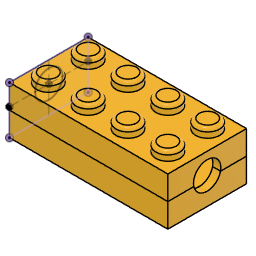
2x4 lego brick 3001 v6 v3 (Autodesk Fusion 360 design; units mm, degrees)
Autodesk Fusion 360 part; units mm, degrees
box "BoxPrimitive1" add length 15.8 width 31.8 height 9.6 placed x (0, 0, -1) y (-1, 0, 0) z (0, 1, 0) at (31.8, 0, 0) makes body 1
box "BoxPrimitive2" add length 13.4 width 29.4 height 8.6 placed x (0, 0, 1) y (1, 0, 0) z (0, 1, 0) at (0, 0, 0) separate body makes body 2
move_body "Move2" bodies 2 to x (1, 0, 0) y (0, 1, 0) z (0, 0, 1) at (1.2, 0, 0)
move_body "Move3" bodies 2 to x (1, 0, 0) y (0, 1, 0) z (0, 0, 1) at (0, 0, -14.6)
combine "Combine1" operation cut target body 1 tool bodies 2
cylinder "CylinderPrimitive1" add diameter 4.8 height 1.8 placed x (1, 0, 0) y (0, 0, -1) z (0, 1, 0) at (0, 9.6, 0) separate body makes body 3
move_body "Move4" bodies 3 to x (1, 0, 0) y (0, 1, 0) z (0, 0, 1) at (3.9, 0, -3.9)
pattern_linear "R-Pattern1" count 4 spacing 8 along (1, 0, 0) count 2 spacing 8 along (0, 0, -1) of bodies 3 makes body 4 at (14.2881, 10.8, -3.661) makes body 5 at (22.2881, 10.8, -3.661) makes body 6 at (30.297, 10.2, -3.7804) makes body 7 at (6.297, 10.2, -11.7804) makes body 8 at (14.297, 10.2, -11.7804) makes body 9 at (22.297, 10.2, -11.7804) makes body 10 at (30.297, 10.2, -11.7804)
combine "Combine3" operation add target body 1 tool bodies 4 10 7 9 8 5 6 3
cylinder "CylinderPrimitive3" add diameter 2.6 height 1.9 placed x (1, 0, 0) y (0, 0, -1) z (0, 1, 0) at (27.9, 11.4, -11.9) separate body makes body 11
pattern_linear "R-Pattern3" count 4 spacing 8 along (-1, 0, 0) count 2 spacing 8 along (0, 0, 1) of bodies 11 makes body 12 at (21.1935, 12.0333, -11.7706) makes body 13 at (13.1935, 12.0333, -11.7706) makes body 14 at (5.1935, 12.0333, -11.7706) makes body 15 at (29.1935, 12.0333, -3.7706) makes body 16 at (21.1935, 12.0333, -3.7706) makes body 17 at (13.1935, 12.0333, -3.7706) makes body 18 at (5.1935, 12.0333, -3.7706)
move_body "Move6" bodies 11 15 13 12 14 16 17 18 to x (1, 0, 0) y (0, 1, 0) z (0, 0, 1) at (0, -3, 0)
combine "Combine4" operation cut target body 1 tool bodies 11 15 13 12 14 16 17 18
sketch "Sketch7" plane through (0, 8.6, 0) normal (0, -1, 0) x (1, 0, 0)
  circle A0 centre (3.9, -3.9) radius 1.3
  circle A1 centre (11.9, -3.9) radius 1.3
  circle A2 centre (19.9, -3.9) radius 1.3
  circle A3 centre (3.9, -11.9) radius 1.3
  circle A4 centre (19.9, -11.9) radius 1.3
  circle A5 centre (11.9, -11.9) radius 1.3
  circle A6 centre (27.9, -3.9) radius 1.3
  circle A7 centre (27.9, -11.9) radius 1.3
  line L0 (30.6, -1.2) -> (1.2, -1.2)
  line L1 (1.2, -1.2) -> (1.2, -14.6)
  line L2 (1.2, -14.6) -> (30.6, -14.6)
  line L3 (30.6, -14.6) -> (30.6, -1.2)
  circle A8 centre (7.9, -7.9) radius 3.255
  line L4 (0, 0) -> (7.9, 0)
  line L5 (0, -7.9) -> (0, 0)
  circle A9 centre (7.9, -7.9) radius 2.4
  dimension "d47" = 6.51
  dimension "d48" = 7.9
  dimension "d49" = 4.8
  constraint horizontal L4
  constraint vertical L5
  constraint coincident L4.start L5.end
  constraint coincident A8.centre A9.centre
  measures "d47" diameter of A8
  measures "d48" distance of L4.start L4.end
  measures "d49" diameter of A9
extrude "Extrude1" add sketch "Sketch7" along normal up to surface (8.6 mm away) separate body contours A8 makes body 19
pattern_linear "R-Pattern4" count 3 spacing 8 along (1, 0, 0) of bodies 19 makes body 20 at (19.1388, 2.8667, -8.2241) makes body 21 at (27.1388, 2.8667, -8.2241)
combine "Combine5" operation add target body 1 tool bodies 20 21 19
sketch "Sketch9" plane through (0, 8.6, 0) normal (0, -1, 0) x (1, 0, 0)
  circle A0 centre (23.9, -7.9) radius 3.255
  line L0 (30.6, -1.2) -> (1.2, -1.2)
  line L1 (1.2, -1.2) -> (1.2, -14.6)
  line L2 (1.2, -14.6) -> (30.6, -14.6)
  line L3 (30.6, -14.6) -> (30.6, -1.2)
  circle A1 centre (27.9, -11.9) radius 1.3
  circle A2 centre (27.9, -3.9) radius 1.3
  circle A3 centre (11.9, -11.9) radius 1.3
  circle A4 centre (19.9, -11.9) radius 1.3
  circle A5 centre (3.9, -11.9) radius 1.3
  circle A6 centre (19.9, -3.9) radius 1.3
  circle A7 centre (11.9, -3.9) radius 1.3
  circle A8 centre (3.9, -3.9) radius 1.3
  circle A9 centre (15.9, -7.9) radius 3.255
  circle A10 centre (7.9, -7.9) radius 3.255
  line L4 (1.2, -14.6) -> (3.9, -14.6)
  line L5 (3.9, -14.6) -> (3.9, -11.9)
  line L6 (3.9, -11.9) -> (1.2, -11.9)
  line L7 (1.2, -11.9) -> (1.2, -14.6)
  line L8 (1.2, -11.9) -> (1.4, -11.9)
  line L9 (1.4, -11.9) -> (1.4, -11.6)
  line L10 (1.4, -11.6) -> (1.2, -11.6)
  line L11 (1.2, -11.6) -> (1.2, -11.9)
  line L12 (1.4, -11.9) -> (1.2, -11.9)
  line L13 (1.2, -11.9) -> (1.2, -12.2)
  line L14 (1.2, -12.2) -> (1.4, -12.2)
  line L15 (1.4, -12.2) -> (1.4, -11.9)
  line L16 (1.2, -11.6) -> (1.4, -11.6)
  line L17 (1.4, -11.6) -> (1.4, -12.2)
  line L18 (1.4, -12.2) -> (1.2, -12.2)
  line L19 (1.2, -12.2) -> (1.2, -11.6)
  line L20 (3.9, -14.6) -> (4.2, -14.6)
  line L21 (4.2, -14.6) -> (4.2, -14.4)
  line L22 (4.2, -14.4) -> (3.9, -14.4)
  line L23 (3.9, -14.4) -> (3.9, -14.6)
  line L24 (3.9, -14.6) -> (3.6, -14.6)
  line L25 (3.6, -14.6) -> (3.6, -14.4)
  line L26 (3.6, -14.4) -> (3.9, -14.4)
  line L27 (3.9, -14.4) -> (3.9, -14.6)
  line L28 (3.6, -14.4) -> (4.2, -14.4)
  line L29 (4.2, -14.4) -> (4.2, -14.6)
  line L30 (4.2, -14.6) -> (3.6, -14.6)
  line L31 (3.6, -14.6) -> (3.6, -14.4)
  line L32 (15.9, -7.9) -> (15.9, -14.6)
  line L33 (15.9, -14.6) -> (16.3, -14.6)
  line L34 (16.3, -14.6) -> (16.3, -11.1349)
  line L35 (16.3, -11.1349) -> (15.9, -11.1349)
  line L36 (15.9, -11.1349) -> (15.9, -14.6)
  line L37 (15.9, -14.6) -> (15.5, -14.6)
  line L38 (15.5, -14.6) -> (15.5, -11.1303)
  line L39 (15.5, -11.1303) -> (15.9, -11.1303)
  line L40 (15.9, -11.1303) -> (15.9, -14.6)
  line L41 (15.9, -7.9) -> (15.9, -1.2)
  line L42 (15.9, -1.2) -> (16.3, -1.2)
  line L43 (16.3, -1.2) -> (16.3, -4.6697)
  line L44 (16.3, -4.6697) -> (15.9, -4.6697)
  line L45 (15.9, -4.6697) -> (15.9, -1.2)
  line L46 (15.9, -1.2) -> (15.5, -1.2)
  line L47 (15.5, -1.2) -> (15.5, -4.6785)
  line L48 (15.5, -4.6785) -> (15.9, -4.6785)
  line L49 (15.9, -4.6785) -> (15.9, -1.2)
  dimension "d58" = 0.3
  dimension "d59" = 0.2
  dimension "d60" = 0.3
  dimension "d67" = 0.3
  dimension "d68" = 0.2
  dimension "d69" = 0.3
  dimension "d76" = 0.4
  dimension "d77" = 0.4
  dimension "d78" = 0.4
  dimension "d79" = 0.4
  constraint horizontal L4
  constraint vertical L5
  constraint horizontal L6
  constraint vertical L7
  constraint coincident A5.centre L5.end
  constraint coincident L1.end L2.start
  constraint horizontal L8
  constraint vertical L9
  constraint horizontal L10
  constraint vertical L11
  constraint horizontal L12
  constraint vertical L13
  constraint horizontal L14
  constraint vertical L15
  constraint horizontal L16
  constraint vertical L17
  constraint horizontal L18
  constraint vertical L19
  constraint horizontal L20
  constraint vertical L21
  constraint horizontal L22
  constraint vertical L23
  constraint horizontal L24
  constraint vertical L25
  constraint horizontal L26
  constraint vertical L27
  constraint horizontal L28
  constraint vertical L29
  constraint horizontal L30
  constraint vertical L31
  constraint coincident A9.centre L32.start
  constraint midpoint L2 L32.end
  constraint horizontal L33
  constraint vertical L34
  constraint horizontal L35
  constraint vertical L36
  constraint horizontal L37
  constraint vertical L38
  constraint horizontal L39
  constraint vertical L40
  constraint coincident A9 L38.end
  constraint midpoint L0 L41.end
  constraint horizontal L42
  constraint vertical L43
  constraint horizontal L44
  constraint vertical L45
  constraint coincident A9 L43.end
  constraint horizontal L46
  constraint vertical L47
  constraint horizontal L48
  constraint vertical L49
  measures "d58" distance of L6.end L10.end
  measures "d59" distance of L6.end L8.end
  measures "d60" distance of L8.end L14.end
  measures "d67" distance of L4.end L20.end
  measures "d68" distance of L4.end L22.end
  measures "d69" distance of L4.end L24.end
  measures "d76" distance of L32.end L33.end
  measures "d77" distance of L32.end L37.end
  measures "d78" distance of L41.end L42.end
  measures "d79" distance of L41.end L46.end
extrude "Extrude5" add sketch "Sketch9" along normal blind 6.3 contours L0 A9 L41 L42 L43 L45 L49 | L0 A9 L41 L45 L46 L47 L49 bodies 1
extrude "Extrude3" add sketch "Sketch9" along normal up to surface (8.6 mm away) separate body contours L2 L5 L20 L21 L22 L23 L27 L28 L29 L30 | L2 L4 L5 L23 L24 L25 L26 L27 L28 L30 L31 makes body 22
extrude "Extrude2" add sketch "Sketch9" along normal up to surface (8.6 mm away) separate body contours L1 L6 L8 L9 L10 L11 L12 L16 L17 L19 | L1 L6 L7 L8 L12 L13 L14 L15 L17 L18 L19 makes body 23
pattern_linear "R-Pattern5" count 2 spacing 8 along (0, 0, 1) count 2 spacing 29.2 along (1, 0, 0) of bodies 23 makes body 24 at (1.2, 5.7333, -3.7) makes body 25 at (30.4, 5.7333, -11.7) makes body 26 at (30.4, 5.7333, -3.7)
pattern_linear "R-Pattern6" count 2 spacing 13.2 along (0, 0, 1) count 4 spacing 8 along (1, 0, 0) of bodies 22 makes body 27 at (3.7, 5.7333, -1.4) makes body 28 at (11.7, 5.7333, -14.6) makes body 29 at (11.7, 5.7333, -1.4) makes body 30 at (19.7, 5.7333, -14.6) makes body 31 at (19.7, 5.7333, -1.4) makes body 32 at (28, 5.7333, -14.6) makes body 33 at (28, 5.7333, -1.4)
combine "Combine6" operation add target body 1 tool bodies 22 25 24 23 26 28 27 29 32 33 30 31
extrude "Extrude4" add sketch "Sketch9" along normal blind 6.3 contours L2 A9 L32 L33 L34 L35 L36 L40 | L2 A9 L32 L36 L37 L38 L40 bodies 1
move_body "Move7" bodies 1 to x (-1, 0, 0) y (0, -1, 0) z (0, 0, 1) at (63.6, 0, 0)
move_body "Move8" bodies 1 to x (-1, 0, 0) y (0, -1, 0) z (0, 0, 1) at (127.2, 0, 0)
sketch "Sketch15" plane through (0, 8.6, 0) normal (0, -1, 0) x (1, 0, 0)
  line L0 (79.1, -1.2) -> (75.8, -1.2)
  line L1 (75.8, -1.2) -> (75.8, -1.4)
  line L2 (75.8, -1.4) -> (75.2, -1.4)
  line L3 (75.2, -1.4) -> (75.2, -1.2)
  line L4 (75.2, -1.2) -> (67.8, -1.2)
  line L5 (67.8, -1.2) -> (67.8, -1.4)
  line L6 (67.8, -1.4) -> (67.2, -1.4)
  line L7 (67.2, -1.4) -> (67.2, -1.2)
  line L8 (67.2, -1.2) -> (64.8, -1.2)
  line L9 (64.8, -1.2) -> (64.8, -3.6)
  line L10 (64.8, -3.6) -> (65, -3.6)
  line L11 (65, -3.6) -> (65, -4.2)
  line L12 (65, -4.2) -> (64.8, -4.2)
  line L13 (64.8, -4.2) -> (64.8, -11.6)
  line L14 (64.8, -11.6) -> (65, -11.6)
  line L15 (65, -11.6) -> (65, -12.2)
  line L16 (65, -12.2) -> (64.8, -12.2)
  line L17 (64.8, -12.2) -> (64.8, -14.6)
  line L18 (64.8, -14.6) -> (67.2, -14.6)
  line L19 (67.2, -14.6) -> (67.2, -14.4)
  line L20 (67.2, -14.4) -> (67.8, -14.4)
  line L21 (67.8, -14.4) -> (67.8, -14.6)
  line L22 (67.8, -14.6) -> (75.2, -14.6)
  line L23 (75.2, -14.6) -> (75.2, -14.4)
  line L24 (95.4, -15.8) -> (63.6, -15.8)
  line L25 (63.6, -15.8) -> (63.6, 0)
  line L26 (63.6, 0) -> (95.4, 0)
  line L27 (95.4, 0) -> (95.4, -15.8)
extrude "Extrude6" add sketch "Sketch15" along normal up to surface (7.9 mm away) from surface at -1 bodies 1
sketch "Sketch17" plane through (63.6, 0, 0) normal (-1, 0, 0) x (0, 0, 1)
  line L0 (0, 0) -> (0, 9.6)
  line L1 (0, 9.6) -> (-15.8, 9.6)
  line L2 (-15.8, 9.6) -> (-15.8, 0)
  line L3 (-15.8, 0) -> (0, 0)
  line L4 (-14.2, 1.6) -> (-1.6, 1.6) construction
  line L5 (-1.6, 1.6) -> (-1.6, 8)
  line L6 (-1.6, 8) -> (-14.2, 8)
  line L7 (-14.2, 8) -> (-14.2, 1.6)
  line L8 (-14.2, 2.7) -> (-1.6, 2.7)
  line L9 (-14.6, 1.7) -> (-14.4, 1.7)
  line L10 (-14.4, 1.7) -> (-14.6, 1.7)
  line L11 (-14.6, 1.7) -> (-14.4, 1.7)
  line L12 (-14.4, 1.7) -> (-14.6, 1.7)
  line L13 (-14.6, 1.7) -> (-14.4, 1.7)
  line L14 (-14.4, 1.7) -> (-14.6, 1.7)
  line L15 (-14.6, 1.7) -> (-14.4, 1.7)
  line L16 (-14.4, 1.7) -> (-14.6, 1.7)
  line L17 (-14.6, 1.7) -> (-12.2, 1.7)
  line L18 (-12.2, 1.7) -> (-11.6, 1.7)
  line L19 (-11.6, 1.7) -> (-4.2, 1.7)
  line L20 (-4.2, 1.7) -> (-3.6, 1.7)
  line L21 (-3.6, 1.7) -> (-1.2, 1.7)
  line L22 (-1.2, 1.7) -> (-1.4, 1.7)
  line L23 (-1.4, 1.7) -> (-1.2, 1.7)
  line L24 (-1.2, 1.7) -> (-1.4, 1.7)
  line L25 (-1.4, 1.7) -> (-1.2, 1.7)
  line L26 (-1.2, 1.7) -> (-1.4, 1.7)
  line L27 (-1.4, 1.7) -> (-1.2, 1.7)
  line L28 (-1.2, 1.7) -> (-1.4, 1.7)
  line L29 (-1.4, 1.7) -> (-1.2, 1.7)
  line L30 (-1.2, 1.7) -> (-3.6, 1.7)
  line L31 (-3.6, 1.7) -> (-4.2, 1.7)
  line L32 (-4.2, 1.7) -> (-11.6, 1.7)
  line L33 (-11.6, 1.7) -> (-12.2, 1.7)
  line L34 (-12.2, 1.7) -> (-14.6, 1.7)
  line L35 (-11.155, 1.7) -> (-4.645, 1.7)
  line L36 (-11.155, 1.7) -> (-4.645, 1.7)
  line L37 (-11.155, 1.7) -> (-4.645, 1.7)
  dimension "d92" = -1.6
  dimension "d93" = 1
  constraint coincident L7 L8.start
  constraint coincident L5 L8.end
  constraint perpendicular L5 L8
  measures "d93" distance of L8 L32
extrude "Extrude8" cut sketch "Sketch17" against normal up to surface (28.6 mm away) from surface at -1.6 contours L5 L6 L7 L8 bodies 1
sketch "Sketch18" plane through (0, 11.4, 0) normal (0, 1, 0) x (-1, 0, 0)
  circle A0 centre (-67.5, -3.9) radius 2.4
  circle A1 centre (-67.5, -11.9) radius 2.4
  circle A2 centre (-75.5, -11.9) radius 2.4
  circle A3 centre (-75.5, -3.9) radius 2.4
  circle A4 centre (-83.5, -3.9) radius 2.4
  circle A5 centre (-83.5, -11.9) radius 2.4
  circle A6 centre (-91.5, -11.9) radius 2.4
  circle A7 centre (-91.5, -3.9) radius 2.4
extrude "Extrude9" add sketch "Sketch18" against normal blind 1.8 bodies 1
ref_plane "WorkPlane1" through (79.5, 4.8, -7.9) normal (0, 1, 0) x (0, 0, -1)
sketch "Sketch19" plane through (63.6, 0, 0) normal (-1, 0, 0) x (0, 0, 1)
  line L0 (-15.8, 9.6) -> (-15.8, 0)
  line L1 (-15.8, 0) -> (0, 0)
  line L2 (0, 0) -> (0, 9.6)
  line L3 (0, 9.6) -> (-15.8, 9.6)
  circle A0 centre (-7.9, 5.4) radius 2.75
  line L4 (-7.9, 9.6) -> (-7.9, 0) construction
  line L5 (0, 5.4) -> (-15.8, 5.4) construction
  dimension "d99" = 5.5
  dimension "d103" = 4.2
  constraint midpoint L3 L4.start
  constraint midpoint L1 L4.end
  constraint midpoint A0.centre L5
  constraint coincident L0 L5.end
  constraint coincident L2 L5.start
  constraint horizontal L5
  measures "d99" diameter of A0
  measures "d103" distance of L3 A0.centre
extrude "Extrude11" cut sketch "Sketch19" against normal up to surface (1.6 mm away) contours A0 bodies 1
extrude "Extrude12" cut sketch "Sketch19" against normal up to surface (1.6 mm away) from surface at -30.2 contours A0 bodies 1
split "Split1" by plane through (79.5, 4.8, -7.9) normal (0, 1, 0) bodies 1 makes body 34 at (84.2667, 8, -5.2028)
fillet "Fillet1" radius 0.7 8 edges at (65.2624, 11.4, -11.0321) (65.2624, 11.4, -3.0321) (73.2624, 11.4, -3.0321) (73.2624, 11.4, -11.0321) (81.2624, 11.4, -11.0321) (81.2624, 11.4, -3.0321) (89.2624, 11.4, -3.0321) (89.2624, 11.4, -11.0321) on bodies 34
named bodies: "bottom", "top"
